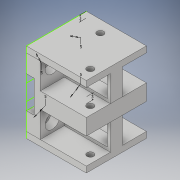
# Autodesk Inventor part: xy 조인트 앞면
Saved by Autodesk Inventor 2018 (Build 220112000, 112)
## iProperties
Created: 2019-01-21
Part Number: xy 조인트 앞면
Material: Generic
Document SubType Name: Modeling
Designer: User
Density: 1 g/cm^3
Appearance: Default
Author: User
Autodesk Inventor part; units mm, degrees
ref_plane "YZ Plane" through (0, 0, 0) normal (1, 0, 0) x (0, 1, 0)
ref_plane "XZ Plane" through (0, 0, 0) normal (0, 1, 0) x (-1, 0, 0)
ref_plane "XY Plane" through (0, 0, 0) normal (0, 0, 1) x (1, 0, 0)
sketch "스케치1" plane through (0, 0, 0) normal (1, 0, 0) x (0, 1, 0)
  line L0 (-17, 15) -> (17, 15)
  line L1 (17, 15) -> (17, -15)
  line L2 (17, -15) -> (-17, -15)
  line L3 (-17, -15) -> (-17, 15)
  circle A0 centre (12, 9) radius 2.5
  circle A1 centre (12, -9) radius 2.5
  circle A2 centre (-12, 9) radius 2.5
  circle A3 centre (-12, -9) radius 2.5
  line L4 (4, 0) -> (4, -15)
  line L5 (4, 0) -> (4, 15)
  line L6 (-4, 0) -> (-4, -15)
  line L7 (-4, 0) -> (-4, 15)
  line L8 (17, -3) -> (8, -3)
  line L9 (17, 3) -> (8, 3)
  line L10 (-8, 3) -> (-17, 3)
  line L11 (-8, -3) -> (-17, -3)
  line L12 (8, -15) -> (8, 15)
  line L13 (-8, -15) -> (-8, 15)
  line L14 (8, -3) -> (4, -3)
  line L15 (8, 3) -> (4, 3)
  line L16 (-4, -3) -> (-8, -3)
  line L17 (-4, 3) -> (-8, 3)
  line L18 (-17, -15) -> (-20, -15)
  line L19 (-20, -15) -> (-20, 15)
  line L20 (-20, 15) -> (-17, 15)
  line L21 (17, -15) -> (20, -15)
  line L22 (20, -15) -> (20, 15)
  line L23 (20, 15) -> (17, 15)
  dimension "d9" = 5
  dimension "d10" = 5
  dimension "d11" = 5
  dimension "d12" = 5
  dimension "d76" = 3
  dimension "d77" = 3
  constraints: 48 end point, 26 point on line, 16 perpendicular, 4 centre point, 2 horizontal, 2 parallel
  measures "d9" diameter of A0
  measures "d10" diameter of A1
  measures "d11" diameter of A2
  measures "d12" diameter of A3
  measures "d76" distance of L2.end L18.end
  measures "d77" distance of L1.end L21.end
extrude "돌출3" add sketch "스케치1" along normal blind 7 contours L0 L13 L10 L3 | L11 L13 L2 L3 | L0 L1 L9 L12 | L8 L1 L2 L12
extrude "돌출4" add sketch "스케치1" along normal blind 30 separate body contours L10 L13 L11 L3 | L17 L7 L6 L16 L13 | L15 L12 L14 L4 L5 | L9 L1 L8 L12
sketch "스케치5" plane through (7, 0, 0) normal (1, 0, 0) x (0, 0, -1)
  circle A0 centre (-9, 12) radius 2.5 projected
  circle A1 centre (-9, 12) radius 3.6
  line L0 (-15, -17) -> (-3, -17) projected
  line L1 (-9, -17) -> (-9, -12)
  circle A2 centre (-9, -12) radius 3.6
  circle A3 centre (9, -12) radius 3.6
  circle A4 centre (9, 12) radius 3.6
  point P0 (0, 0)
  dimension "d63" = 7.2
  dimension "d64" = 5
  dimension "d65" = 7.2
  dimension "d66" = 7.2
  dimension "d67" = 7.2
  constraints: 4 centre point, 2 coincident, 2 end point, 1 midpoint, 1 vertical
  measures "d63" diameter of A1
  measures "d64" distance of L1.start L1.end
  measures "d65" diameter of A2
  measures "d66" diameter of A3
  measures "d67" diameter of A4
extrude "돌출12" cut sketch "스케치5" against normal blind 4.2 bodies 1
extrude "돌출13" add sketch "스케치1" along normal blind 7 contours L0 L7 L17 L13 | L17 L7 L6 L16 L13 | L0 L12 L15 L5 | L16 L6 L2 L13 | L15 L12 L14 L4 L5 | L12 L2 L4 L14 bodies 1
extrude "돌출14" add sketch "스케치1" along normal blind 30 contours L0 L5 L4 L2 L6 L7 bodies 1
extrude "돌출15" cut sketch "스케치1" along normal blind 4 contours L0 L7 L17 L13 | L0 L5 L4 L2 L6 L7 | L17 L7 L6 L16 L13 | L0 L12 L15 L5 | L16 L6 L2 L13 | L15 L12 L14 L4 L5 | L12 L2 L4 L14 bodies 1 2
extrude "돌출16" add sketch "스케치1" along normal blind 30 contours L3 L18 L19 L20 | L23 L22 L21 L1 bodies 2
sketch "스케치6" plane through (0, 20, 15) normal (0, 1, 0) x (1, 0, 0)
  line L0 (0, 15) -> (13, 15)
  line L1 (13, 15) -> (13, 24)
  line L2 (13, 24) -> (26, 24)
  line L3 (26, 24) -> (26, 6)
  circle A0 centre (13, 24) radius 1.65
  circle A1 centre (26, 6) radius 1.65
  dimension "d80" = 13
  dimension "d81" = 9
  dimension "d83" = 13
  dimension "d84" = 18
  dimension "d85" = 3.3
  dimension "d86" = 3.3
  constraints: 8 end point, 2 centre point, 2 coincident, 2 horizontal, 1 perpendicular, 1 vertical
  measures "d80" distance of L0.start L0.end
  measures "d81" distance of L0.end L1.end
  measures "d83" distance of L1.end L2.end
  measures "d84" distance of L2.end L3.end
  measures "d85" diameter of A0
  measures "d86" diameter of A1
extrude "돌출17" cut sketch "스케치6" against normal blind 40 bodies 2 1
sketch "스케치7" plane through (30, 4, -3) normal (0, 0, -1) x (-1, 0, 0)
  line L0 (0, 16) -> (0, 13) projected
  line L1 (23, 0) -> (23, 13) projected
  line L2 (23, 4) -> (23, 13) projected
  line L3 (23, 0) -> (0, 0) projected
  line L4 (30, 13) -> (0, 13) projected
  line L5 (0, 13) -> (1.5, 13)
  line L6 (1.5, 13) -> (1.5, 11.5)
  line L7 (23, 0) -> (21.5, 0)
  line L8 (26, 0) -> (0, 0) projected
  line L9 (21.5, 0) -> (21.5, 1.5)
  line L10 (1.5, 11.5) -> (21.5, 11.5)
  line L11 (21.5, 11.5) -> (21.5, 1.5)
  line L12 (21.5, 1.5) -> (1.5, 1.5)
  line L13 (1.5, 1.5) -> (1.5, 11.5)
  line L14 (23, -8) -> (0, -8) projected
  line L15 (0, -8) -> (1.5, -8)
  line L16 (1.5, -8) -> (1.5, -9.5)
  line L17 (30, -21) -> (0, -21) projected
  line L18 (23, -21) -> (21.5, -21)
  line L19 (21.5, -21) -> (21.5, -19.5)
  line L20 (1.5, -9.5) -> (21.5, -9.5)
  line L21 (21.5, -9.5) -> (21.5, -19.5)
  line L22 (21.5, -19.5) -> (1.5, -19.5)
  line L23 (1.5, -19.5) -> (1.5, -9.5)
  point P0 (30, -4)
  dimension "d89" = 1.5
  dimension "d90" = 1.5
  dimension "d91" = 1.5
  dimension "d92" = 1.5
  dimension "d93" = 1.5
  dimension "d94" = 1.5
  dimension "d95" = 1.5
  dimension "d96" = 1.5
  constraints: 32 end point, 6 perpendicular, 5 point on line, 4 parallel, 2 horizontal
  measures "d89" distance of L0.end L5.end
  measures "d90" distance of L5.end L6.end
  measures "d91" distance of L1.start L7.end
  measures "d92" distance of L7.end L9.end
  measures "d93" distance of L14.end L15.end
  measures "d94" distance of L15.end L16.end
  measures "d95" distance of L18.start L18.end
  measures "d96" distance of L18.end L19.end
extrude "돌출18" cut sketch "스케치7" against normal blind 10 contours L12 L13 L10 L11 | L20 L21 L22 L23 bodies 2
